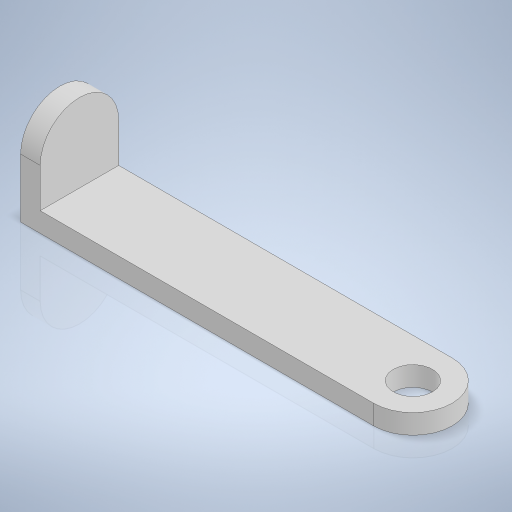
# Autodesk Inventor part: 1 part 11
Saved by Autodesk Inventor 2024 (Build 280153000, 153)
## iProperties
Created: 2024-07-30
Part Number: 1 part 11
Material: Generisch
Document SubType Name: Modeling
Designer: ffogue
Density: 1 g/cm^3
Appearance: Vorgabe
Author: ffogue
Autodesk Inventor part; units mm, degrees
ref_plane "YZ Plane" through (0, 0, 0) normal (1, 0, 0) x (0, 1, 0)
ref_plane "XZ Plane" through (0, 0, 0) normal (0, 1, 0) x (-1, 0, 0)
ref_plane "XY Plane" through (0, 0, 0) normal (0, 0, 1) x (1, 0, 0)
sketch "Skizze1" plane through (0, 0, 0) normal (0, 0, 1) x (1, 0, 0)
  arc A0 (0, -3) -> (0, 3) centre (0, 0) ccw
  line L0 (0, 3) -> (-25.5, 3)
  line L1 (-25.5, 3) -> (-25.5, -3)
  line L2 (-25.5, -3) -> (0, -3)
  dimension "d0" = 3
  dimension "d1" = 25.5
  constraints: 6 end point, 2 perpendicular, 2 point on circle, 2 vertical alignment, 1 centre point, 1 coincident, 1 horizontal
  measures "d0" radius of A0
  measures "d1" distance from line of point (0, 0) L1
extrude "Extrusion1" add sketch "Skizze1" along normal blind 1.5
sketch "Skizze3" plane through (-25.5, -3, 0) normal (-1, 0, 0) x (0, 0, 1)
  line L0 (0, 6) -> (0, 0) projected
  line L1 (0, 0) -> (1.5, 0) projected
  line L2 (1.5, 6) -> (1.5, 0) projected
  line L3 (0, 6) -> (1.5, 6) projected
  line L4 (0, 6) -> (4.5, 6)
  arc A0 (4.5, 0) -> (4.5, 6) centre (4.5, 3) ccw
  line L5 (4.5, 0) -> (0, 0)
  point P0 (0, 3)
  point P1 (7.5, 3)
  dimension "d4" = 7.5
  constraints: 4 end point, 3 point on circle, 2 tangent, 1 centre point, 1 collinear, 1 horizontal
  measures "d4" distance from line of L0 point (7.5, 3)
extrude "Extrusion2" add sketch "Skizze3" along normal blind 1.5
sketch "Skizze4" plane through (0, 0, 1.5) normal (0, 0, 1) x (1, 0, 0)
  arc A0 (0, -3) -> (0, 3) centre (0, 0) ccw projected
  constraints: 1 coincident
hole "Bohrung1" at (0, 0, 1.5) direction (0, 0, -1) diameter 3 depth 1.5
